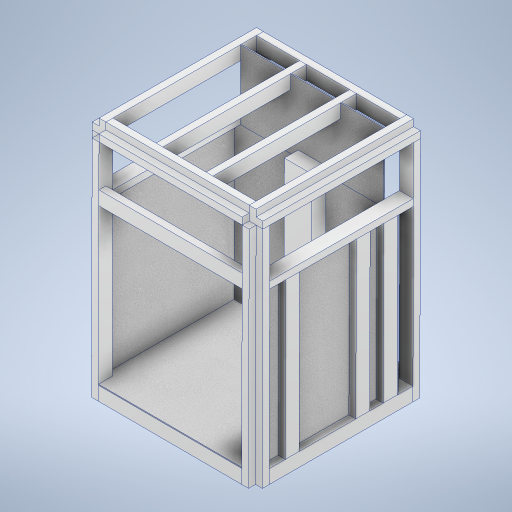
# Autodesk Inventor part: Rev IV Envelope Frame Study
Saved by Autodesk Inventor 2024 (Build 280153000, 153)
## iProperties
Created: 2024-12-08
Part Number: Rev IV Envelope Frame Study
Material: Aluminum 6061
Document SubType Name: Modeling
Designer: Ishaan
Density: 2.7 g/cm^3
Appearance: Aluminum - Flat
Author: Ishaan
Autodesk Inventor part; units mm, degrees
ref_plane "YZ Plane" through (0, 0, 0) normal (1, 0, 0) x (0, 1, 0)
ref_plane "XZ Plane" through (0, 0, 0) normal (0, 1, 0) x (-1, 0, 0)
ref_plane "XY Plane" through (0, 0, 0) normal (0, 0, 1) x (1, 0, 0)
sketch "Sketch1" plane through (0, 0, 0) normal (0, 0, 1) x (1, 0, 0)
  line L0 (247.5, -247.5) -> (-247.5, -247.5) construction
  line L1 (-247.5, -247.5) -> (-247.5, 247.5) construction
  line L2 (-247.5, 247.5) -> (247.5, 247.5) construction
  line L3 (247.5, 247.5) -> (247.5, -247.5) construction
  line L4 (247.5, -247.5) -> (-247.5, 247.5) construction
  line L5 (-247.5, -247.5) -> (247.5, 247.5) construction
  line L6 (-247.5, 247.5) -> (-207.5, 247.5)
  line L7 (-207.5, 247.5) -> (-207.5, 207.5)
  line L8 (-207.5, 207.5) -> (-247.5, 207.5)
  line L9 (-247.5, 207.5) -> (-247.5, 247.5)
  line L10 (-247.5, 247.5) -> (-227.5, 247.5)
  line L11 (-227.5, 247.5) -> (-227.5, 227.5)
  line L12 (-227.5, 227.5) -> (-247.5, 227.5)
  line L13 (-247.5, 227.5) -> (-247.5, 247.5)
  line L14 (247.5, 247.5) -> (207.5, 247.5)
  line L15 (207.5, 247.5) -> (207.5, 207.5)
  line L16 (207.5, 207.5) -> (247.5, 207.5)
  line L17 (247.5, 207.5) -> (247.5, 247.5)
  line L18 (247.5, 247.5) -> (227.5, 247.5)
  line L19 (227.5, 247.5) -> (227.5, 227.5)
  line L20 (227.5, 227.5) -> (247.5, 227.5)
  line L21 (247.5, 227.5) -> (247.5, 247.5)
  line L22 (247.5, -247.5) -> (207.5, -247.5)
  line L23 (207.5, -247.5) -> (207.5, -207.5)
  line L24 (207.5, -207.5) -> (247.5, -207.5)
  line L25 (247.5, -207.5) -> (247.5, -247.5)
  line L26 (247.5, -247.5) -> (227.5, -247.5)
  line L27 (227.5, -247.5) -> (227.5, -227.5)
  line L28 (227.5, -227.5) -> (247.5, -227.5)
  line L29 (247.5, -227.5) -> (247.5, -247.5)
  line L30 (-247.5, -247.5) -> (-207.5, -247.5)
  line L31 (-207.5, -247.5) -> (-207.5, -207.5)
  line L32 (-207.5, -207.5) -> (-247.5, -207.5)
  line L33 (-247.5, -207.5) -> (-247.5, -247.5)
  line L34 (-247.5, -247.5) -> (-227.5, -247.5)
  line L35 (-227.5, -247.5) -> (-227.5, -227.5)
  line L36 (-227.5, -227.5) -> (-247.5, -227.5)
  line L37 (-247.5, -227.5) -> (-247.5, -247.5)
  point P0 (0, 0)
  point P1 (227.5, -247.5)
  point P2 (247.5, -227.5)
  point P3 (247.5, 227.5)
  point P4 (227.5, 247.5)
  point P5 (-247.5, -227.5)
  point P6 (-227.5, -247.5)
  point P7 (-227.5, 247.5)
  point P8 (-247.5, 227.5)
  dimension "d0" = 495
  dimension "d1" = 495
  dimension "d2" = 40
  dimension "d3" = 40
  dimension "d4" = 20
  dimension "d5" = 20
  dimension "d6" = 40
  dimension "d7" = 40
  dimension "d8" = 20
  dimension "d9" = 20
  dimension "d10" = 40
  dimension "d11" = 40
  dimension "d12" = 20
  dimension "d13" = 20
  dimension "d14" = 40
  dimension "d15" = 40
  dimension "d16" = 20
  dimension "d17" = 20
  constraints: 76 end point, 18 parallel, 9 horizontal, 9 perpendicular, 2 midpoint
  measures "d0" distance of L1.end L2.end
  measures "d1" distance of L0.end L1.end
  measures "d2" distance of L7.end L8.end
  measures "d3" distance of L6.end L7.end
  measures "d4" distance of L11.end L12.end
  measures "d5" distance of L10.end L11.end
  measures "d6" distance of L16.end L15.end
  measures "d7" distance of L15.end L14.end
  measures "d8" distance of L20.end L19.end
  measures "d9" distance of L19.end L18.end
  measures "d10" distance of L23.end L24.end
  measures "d11" distance of L22.end L23.end
  measures "d12" distance of L27.end L28.end
  measures "d13" distance of L26.end L27.end
  measures "d14" distance of L32.end L31.end
  measures "d15" distance of L31.end L30.end
  measures "d16" distance of L36.end L35.end
  measures "d17" distance of L35.end L34.end
extrude "Extrusion1" add sketch "Sketch1" along normal blind 650 contours L6 L7 L8 L9 L12 L11 | L19 L20 L17 L16 L15 L14 | L22 L23 L24 L25 L28 L27 | L35 L36 L33 L32 L31 L30
sketch "Sketch2" plane through (-247.5, 227.5, 0) normal (0, 1, 0) x (1, 0, 0)
  line L0 (20, 0) -> (0, 0) projected
  line L1 (0, 0) -> (0, -650) projected
  line L2 (20, -650) -> (0, -650) projected
  line L3 (20, 0) -> (20, -650) projected
  line L4 (0, -650) -> (40, -650) projected
  line L5 (0, -650) -> (40, -650)
  line L6 (40, -650) -> (40, -690)
  line L7 (40, -690) -> (0, -690)
  line L8 (0, -690) -> (0, -650)
  line L9 (0, -690) -> (20, -690)
  line L10 (20, -690) -> (20, -670)
  line L11 (20, -670) -> (0, -670)
  line L12 (0, -670) -> (0, -690)
  line L13 (495, 0) -> (495, -650) projected
  line L14 (495, -650) -> (455, -650)
  line L15 (455, -650) -> (455, -690)
  line L16 (455, -690) -> (495, -690)
  line L17 (495, -690) -> (495, -650)
  line L18 (495, -690) -> (475, -690)
  line L19 (475, -690) -> (475, -670)
  line L20 (475, -670) -> (495, -670)
  line L21 (495, -670) -> (495, -690)
  point P0 (247.5, 0)
  point P1 (0, -670)
  dimension "d20" = 40
  dimension "d21" = 40
  dimension "d22" = 20
  dimension "d23" = 20
  dimension "d24" = 40
  dimension "d25" = 40
  dimension "d26" = 20
  dimension "d27" = 20
  constraints: 32 end point, 8 parallel, 4 horizontal, 4 perpendicular
  measures "d20" distance of L6.end L7.end
  measures "d21" distance of L5.end L6.end
  measures "d22" distance of L11.end L10.end
  measures "d23" distance of L10.end L9.end
  measures "d24" distance of L16.end L15.end
  measures "d25" distance of L15.end L14.end
  measures "d26" distance of L19.end L20.end
  measures "d27" distance of L18.end L19.end
extrude "Extrusion2" add sketch "Sketch2" against normal up to surface (455 mm away) separate body contours L4 L6 L7 L10 L11 L8 L2 | L17 L20 L19 L16 L15 L14
sketch "Sketch3" plane through (-207.5, 227.5, 690) normal (1, 0, 0) x (0, 0, -1)
  line L0 (0, -455) -> (40, -455) projected
  line L1 (40, 0) -> (40, -455) projected
  line L2 (0, 0) -> (40, 0) projected
  line L3 (0, 0) -> (0, -455) projected
  line L4 (40, -475) -> (40, -435) projected
  line L5 (40, -475) -> (0, -475)
  line L6 (0, -475) -> (0, -435)
  line L7 (0, -435) -> (40, -435)
  line L8 (40, -435) -> (40, -475)
  line L9 (0, -475) -> (20, -475)
  line L10 (20, -475) -> (20, -455)
  line L11 (20, -455) -> (0, -455)
  line L12 (0, -455) -> (0, -475)
  line L13 (40, -20) -> (40, 20) projected
  line L14 (690, 20) -> (40, 20) projected
  line L15 (40, 20) -> (0, 20)
  line L16 (0, 20) -> (0, -20)
  line L17 (0, -20) -> (40, -20)
  line L18 (40, -20) -> (40, 20)
  line L19 (0, 20) -> (20, 20)
  line L20 (20, 20) -> (20, 0)
  line L21 (20, 0) -> (0, 0)
  line L22 (0, 0) -> (0, 20)
  point P0 (690, -227.5)
  point P1 (20, -455)
  point P2 (0, -435)
  dimension "d30" = 40
  dimension "d31" = 40
  dimension "d32" = 20
  dimension "d33" = 20
  dimension "d34" = 40
  dimension "d35" = 40
  dimension "d36" = 20
  dimension "d37" = 20
  constraints: 32 end point, 8 parallel, 4 horizontal, 4 perpendicular
  measures "d30" distance of L6.end L7.end
  measures "d31" distance of L5.end L6.end
  measures "d32" distance of L11.end L10.end
  measures "d33" distance of L10.end L9.end
  measures "d34" distance of L17.end L16.end
  measures "d35" distance of L16.end L15.end
  measures "d36" distance of L20.end L21.end
  measures "d37" distance of L19.end L20.end
extrude "Extrusion3" add sketch "Sketch3" along normal up to surface (415 mm away) separate body contours L3 L7 L1 L0 | L0 L4 L5 L10 | L3 L2 L1 L17 | L20 L15 L13 L2
sketch "Sketch4" plane through (207.5, 207.5, 0) normal (0, -1, 0) x (1, 0, 0)
  line L0 (-455, 0) -> (-415, 0) projected
  line L1 (-415, 0) -> (-415, 650) projected
  line L2 (-455, 650) -> (-415, 650) projected
  line L3 (-455, 0) -> (-455, 650) projected
  line L4 (0, 0) -> (40, 0) projected
  line L5 (40, 0) -> (40, 650) projected
  line L6 (0, 650) -> (40, 650) projected
  line L7 (0, 0) -> (0, 650) projected
  line L8 (-455, 0) -> (-415, 0)
  line L9 (-415, 0) -> (-415, 40)
  line L10 (-415, 40) -> (-455, 40)
  line L11 (-455, 40) -> (-455, 0)
  line L12 (40, 0) -> (0, 0)
  line L13 (0, 0) -> (0, 40)
  line L14 (0, 40) -> (40, 40)
  line L15 (40, 40) -> (40, 0)
  point P0 (-207.5, 0)
  dimension "d40" = 40
  dimension "d41" = 40
  dimension "d42" = 40
  dimension "d43" = 40
  constraints: 16 end point, 4 parallel, 2 horizontal, 2 perpendicular
  measures "d40" distance of L10.end L9.end
  measures "d41" distance of L9.end L8.end
  measures "d42" distance of L13.end L14.end
  measures "d43" distance of L12.end L13.end
extrude "Extrusion4" add sketch "Sketch4" along normal up to surface (415 mm away) separate body contours L3 L10 L1 L0 | L7 L14 L5 L4
sketch "Sketch5" plane through (-207.5, -247.5, 0) normal (1, 0, 0) x (0, 0, -1)
  line L0 (0, 0) -> (0, 40) projected
  line L1 (-650, 0) -> (-650, 40) projected
  line L2 (0, 0) -> (-650, 0) projected
  line L3 (0, 455) -> (0, 495) projected
  line L4 (0, 495) -> (-650, 495) projected
  line L5 (-650, 455) -> (-650, 495) projected
  line L6 (0, 0) -> (-40, 0)
  line L7 (-40, 0) -> (-40, 20)
  line L8 (-40, 20) -> (0, 20)
  line L9 (0, 20) -> (0, 0)
  line L10 (0, 495) -> (-40, 495)
  line L11 (-40, 495) -> (-40, 475)
  line L12 (-40, 475) -> (0, 475)
  line L13 (0, 475) -> (0, 495)
  line L14 (-40, 455) -> (-40, 40) projected
  point P0 (0, 247.5)
  point P1 (0, 475)
  point P2 (0, 20)
  dimension "d91" = 20
  dimension "d111" = 20
  constraints: 16 end point, 4 parallel, 2 collinear, 2 horizontal, 2 perpendicular
  measures "d91" distance of L10.end L11.end
  measures "d111" distance of L6.end L7.end
extrude "Extrusion5" add sketch "Sketch5" along normal up to surface (415 mm away) separate body
sketch "Sketch6" plane through (-247.5, 207.5, 40) normal (0, 0, 1) x (1, 0, 0)
  line L0 (495, 0) -> (455, 0) projected
  line L1 (455, 0) -> (455, 40) projected
  line L2 (455, 40) -> (475, 40) projected
  line L3 (475, 40) -> (475, 20) projected
  line L4 (475, 20) -> (495, 20) projected
  line L5 (495, 20) -> (495, 0) projected
  line L6 (0, -415) -> (40, -415) projected
  line L7 (40, -435) -> (40, -455) projected
  line L8 (40, -455) -> (20, -455) projected
  line L9 (20, -455) -> (20, -435) projected
  line L10 (20, -435) -> (0, -435) projected
  line L11 (0, -435) -> (0, -415) projected
  line L12 (455, -415) -> (495, -415) projected
  line L13 (495, -415) -> (495, -435) projected
  line L14 (495, -435) -> (475, -435) projected
  line L15 (475, -435) -> (475, -455) projected
  line L16 (475, -455) -> (455, -455) projected
  line L17 (455, -455) -> (455, -415) projected
  line L18 (40, 0) -> (0, 0) projected
  line L19 (0, 0) -> (0, 20) projected
  line L20 (0, 20) -> (20, 20) projected
  line L21 (20, 20) -> (20, 40) projected
  line L22 (20, 40) -> (40, 40) projected
  line L23 (40, 40) -> (40, 20) projected
  line L24 (455, -415) -> (455, 0) projected
  line L25 (455, 0) -> (495, 0) projected
  line L26 (495, 0) -> (495, -415) projected
  line L27 (495, -415) -> (455, -415) projected
  line L28 (0, 0) -> (40, 0) projected
  line L29 (40, 20) -> (40, -435) projected
  line L30 (40, -415) -> (0, -415) projected
  line L31 (0, -415) -> (0, 0) projected
  line L32 (455, 20) -> (40, 20) projected
  line L33 (40, 20) -> (40, 40) projected
  line L34 (40, 40) -> (455, 40) projected
  line L35 (455, 40) -> (455, 20) projected
  line L36 (40, -455) -> (40, -435) projected
  line L37 (40, -435) -> (455, -435) projected
  line L38 (455, -435) -> (455, -455) projected
  line L39 (455, -455) -> (40, -455) projected
  line L40 (0, -369) -> (20, -369)
  line L41 (20, -369) -> (20, -329)
  line L42 (20, -329) -> (0, -329)
  line L43 (0, -329) -> (0, -369)
  line L44 (20, -165) -> (0, -165)
  line L45 (0, -165) -> (0, -125)
  line L46 (0, -125) -> (20, -125)
  line L47 (20, -125) -> (20, -165)
  line L48 (0, -46) -> (20, -46)
  line L49 (20, -46) -> (20, -86)
  line L50 (20, -86) -> (0, -86)
  line L51 (0, -86) -> (0, -46)
  line L52 (10, -165) -> (10, -329) construction
  point P0 (247.5, -207.5)
  point P1 (0, -369)
  point P2 (0, -46)
  point P3 (10, -247)
  dimension "d48" = 20
  dimension "d49" = 40
  dimension "d50" = 20
  dimension "d51" = 40
  dimension "d52" = 20
  dimension "d53" = 40
  dimension "d54" = 86
  dimension "d57" = 86
  dimension "d128" = 208
  dimension "d129" = 164
  constraints: 26 end point, 6 parallel, 3 horizontal, 3 midpoint, 3 perpendicular, 2 point on line, 1 collinear
  measures "d48" distance of L42.end L41.end
  measures "d49" distance of L41.end L40.end
  measures "d50" distance of L45.end L46.end
  measures "d51" distance of L44.end L45.end
  measures "d52" distance of L49.end L50.end
  measures "d53" distance of L48.end L49.end
  measures "d54" distance between parallel lines of L42 L6
  measures "d57" distance between parallel lines of L28 L50
  measures "d128" distance from line of L39 point (10, -247)
  measures "d129" distance of L52.start L52.end
extrude "Extrusion6" add sketch "Sketch6" along normal blind 450 separate body contours L48 L49 L50 L31 | L31 L42 L41 L40 | L46 L47 L44 L31
mirror "Mirror1" about plane through (0, 0, 0) normal (1, 0, 0) of "Extrusion6" bodies 6
sketch "Sketch7" plane through (-247.5, 207.5, 0) normal (0, -1, 0) x (1, 0, 0)
  line L0 (0, 0) -> (40, 0) projected
  line L1 (40, 0) -> (40, 650) projected
  line L2 (0, 650) -> (40, 650) projected
  line L3 (0, 0) -> (0, 650) projected
  line L4 (455, 0) -> (495, 0) projected
  line L5 (495, 0) -> (495, 650) projected
  line L6 (455, 650) -> (495, 650) projected
  line L7 (455, 0) -> (455, 650) projected
  line L8 (0, 490) -> (40, 490)
  line L9 (40, 490) -> (40, 510)
  line L10 (40, 510) -> (0, 510)
  line L11 (0, 510) -> (0, 490)
  line L12 (495, 490) -> (455, 490)
  line L13 (455, 490) -> (455, 510)
  line L14 (455, 510) -> (495, 510)
  line L15 (495, 510) -> (495, 490)
  line L16 (40, 0) -> (40, 650) projected
  point P0 (247.5, 0)
  point P1 (0, 510)
  dimension "d60" = 20
  constraints: 16 end point, 4 parallel, 2 collinear, 2 horizontal, 2 perpendicular, 1 point on line
  measures "d60" distance of L9.end L8.end
extrude "Extrusion7" add sketch "Sketch7" along normal up to surface (415 mm away) separate body contours L3 L10 L1 L8 | L7 L14 L5 L12
sketch "Sketch8" plane through (-207.5, -247.5, 0) normal (1, 0, 0) x (0, 0, -1)
  line L0 (0, 0) -> (0, 40) projected
  line L1 (0, 40) -> (-650, 40) projected
  line L2 (-650, 0) -> (-650, 40) projected
  line L3 (0, 0) -> (-650, 0) projected
  line L4 (0, 0) -> (-650, 0) projected
  line L5 (-490, 0) -> (-530, 0)
  line L6 (-530, 0) -> (-530, 20)
  line L7 (-530, 20) -> (-490, 20)
  line L8 (-490, 20) -> (-490, 0)
  line L9 (-490, 455) -> (-490, 40) projected
  point P0 (0, 247.5)
  dimension "d64" = 40
  dimension "d65" = 20
  constraints: 8 end point, 2 parallel, 1 collinear, 1 horizontal, 1 perpendicular, 1 point on line
  measures "d64" distance of L6.end L7.end
  measures "d65" distance of L5.end L6.end
extrude "Extrusion8" add sketch "Sketch8" along normal up to surface (415 mm away) separate body contours L3 L6 L7 L8
sketch "Sketch12" plane through (-227.5, -161.5, 40) normal (1, 0, 0) x (0, 0, -1)
  line L0 (-450, 369) -> (-450, -46) projected
  line L1 (0, 323) -> (-450, 323) projected
  line L2 (0, 283) -> (0, 323) projected
  line L3 (0, 323) -> (-450, 323)
  line L4 (-450, 323) -> (-450, -46)
  line L5 (-450, -46) -> (0, -46)
  line L6 (0, -46) -> (0, 323)
  point P0 (40, 161.5)
  constraints: 8 end point, 2 parallel, 1 horizontal, 1 perpendicular
extrude "Extrusion12" add sketch "Sketch12" along normal blind 3 separate body
mirror "Mirror2" about plane through (0, 0, 0) normal (1, 0, 0) of "Extrusion12" bodies 9
sketch "Sketch16" plane through (-207.5, 227.5, 40) normal (0, 0, 1) x (1, 0, 0)
  line L0 (415, 20) -> (415, 0) projected
  line L1 (0, 20) -> (415, 20) projected
  line L2 (0, 20) -> (0, 0) projected
  line L3 (0, 0) -> (415, 0) projected
  line L4 (290, -23) -> (270, -23)
  line L5 (270, -23) -> (270, -63)
  line L6 (270, -63) -> (290, -63)
  line L7 (290, -63) -> (290, -23)
  line L8 (145, -23) -> (125, -23)
  line L9 (125, -23) -> (125, -63)
  line L10 (125, -63) -> (145, -63)
  line L11 (145, -63) -> (145, -23)
  line L12 (270, -43) -> (145, -43) construction
  point P0 (207.5, -227.5)
  point P1 (207.5, -43)
  point P2 (125, 20)
  point P3 (270, 20)
  point P4 (125, 0)
  point P5 (145, 0)
  point P6 (270, 0)
  point P7 (290, 0)
  dimension "d99" = 20
  dimension "d100" = 40
  dimension "d101" = 20
  dimension "d102" = 40
  dimension "d103" = 125
  dimension "d104" = 125
  dimension "d127" = 83
  constraints: 18 end point, 4 parallel, 3 midpoint, 2 horizontal, 2 perpendicular, 1 collinear, 1 vertical alignment
  measures "d99" distance of L6.end L5.end
  measures "d100" distance of L5.end L4.end
  measures "d101" distance of L10.end L9.end
  measures "d102" distance of L9.end L8.end
  measures "d103" distance of L12.start L12.end
  measures "d104" distance between parallel lines of L0 L7
  measures "d127" distance between parallel lines of L6 L1
extrude "Extrusion16" add sketch "Sketch16" along normal up to surface (610 mm away) separate body contours L7 L6 L5 L4 | L11 L10 L9 L8
sketch "Sketch17" plane through (-207.5, 207.5, 650) normal (0, -1, 0) x (1, 0, 0)
  line L0 (125, 0) -> (145, 0) projected
  line L1 (270, 0) -> (290, 0) projected
  line L2 (415, 40) -> (415, 0) projected
  line L3 (0, 40) -> (415, 40) projected
  line L4 (0, 40) -> (0, 0) projected
  line L5 (0, 0) -> (415, 0) projected
  line L6 (125, 0) -> (145, 0)
  line L7 (145, 0) -> (145, 40)
  line L8 (145, 40) -> (125, 40)
  line L9 (125, 40) -> (125, 0)
  line L10 (290, 0) -> (270, 0)
  line L11 (270, 0) -> (270, 40)
  line L12 (270, 40) -> (290, 40)
  line L13 (290, 40) -> (290, 0)
  point P0 (207.5, -650)
  point P1 (290, 40)
  point P2 (125, 40)
  constraints: 16 end point, 4 parallel, 4 point on line, 2 horizontal, 2 perpendicular
extrude "Extrusion17" add sketch "Sketch17" along normal up to surface (415 mm away) separate body contours L9 L3 L7 L0 | L11 L3 L13 L1
sketch "Sketch18" plane through (-207.5, 227.5, 0) normal (0, -1, 0) x (1, 0, 0)
  line L0 (125, 40) -> (145, 40) projected
  line L1 (145, 40) -> (125, 40) projected
  line L2 (290, 40) -> (270, 40) projected
  line L3 (270, 40) -> (290, 40) projected
  line L4 (0, 0) -> (415, 0) projected
  line L5 (125, 40) -> (145, 40)
  line L6 (145, 40) -> (145, 0)
  line L7 (145, 0) -> (125, 0)
  line L8 (125, 0) -> (125, 40)
  line L9 (290, 40) -> (270, 40)
  line L10 (270, 40) -> (270, 0)
  line L11 (270, 0) -> (290, 0)
  line L12 (290, 0) -> (290, 40)
  point P0 (207.5, 0)
  point P1 (270, 0)
  point P2 (125, 40)
  point P3 (125, 0)
  point P4 (145, 40)
  constraints: 16 end point, 4 parallel, 4 point on line, 2 horizontal, 2 perpendicular
extrude "Extrusion18" add sketch "Sketch18" along normal up to surface (455 mm away) separate body
sketch "Sketch19" plane through (-247.5, 161.5, 40) normal (0, 1, 0) x (1, 0, 0)
  line L0 (455, -610) -> (495, -610) projected
  line L1 (495, -610) -> (495, -630) projected
  line L2 (495, -630) -> (475, -630) projected
  line L3 (475, -630) -> (475, -650) projected
  line L4 (475, -650) -> (455, -650) projected
  line L5 (455, -650) -> (455, -610) projected
  line L6 (20, -650) -> (20, -630) projected
  line L7 (20, -630) -> (0, -630) projected
  line L8 (0, -630) -> (0, -610) projected
  line L9 (0, -610) -> (40, -610) projected
  line L10 (40, -610) -> (40, -650) projected
  line L11 (40, -650) -> (20, -650) projected
  line L12 (455, 0) -> (455, 40) projected
  line L13 (455, 40) -> (495, 40) projected
  line L14 (495, 40) -> (495, 0) projected
  line L15 (495, 0) -> (455, 0) projected
  line L16 (0, 40) -> (40, 40) projected
  line L17 (40, 40) -> (40, 0) projected
  line L18 (40, 0) -> (0, 0) projected
  line L19 (0, 0) -> (0, 40) projected
  line L20 (0, -450) -> (0, 0) projected
  line L21 (0, 0) -> (20, 0) projected
  line L22 (20, 0) -> (20, -450) projected
  line L23 (20, -450) -> (0, -450) projected
  line L24 (495, 0) -> (495, -450) projected
  line L25 (495, -450) -> (475, -450) projected
  line L26 (475, -450) -> (475, 0) projected
  line L27 (475, 0) -> (495, 0) projected
  line L28 (455, -470) -> (455, -450) projected
  line L29 (455, -450) -> (495, -450) projected
  line L30 (495, -450) -> (495, -470) projected
  line L31 (495, -470) -> (455, -470) projected
  line L32 (0, -450) -> (40, -450) projected
  line L33 (40, -450) -> (40, -470) projected
  line L34 (40, -470) -> (0, -470) projected
  line L35 (0, -470) -> (0, -450) projected
  line L36 (23, -450) -> (20, -450) projected
  line L37 (20, -450) -> (20, 0) projected
  line L38 (20, 0) -> (23, 0) projected
  line L39 (23, 0) -> (23, -450) projected
  line L40 (475, -450) -> (472, -450) projected
  line L41 (472, -450) -> (472, 0) projected
  line L42 (472, 0) -> (475, 0) projected
  line L43 (475, 0) -> (475, -450) projected
  line L44 (330, -650) -> (310, -650) projected
  line L45 (310, -650) -> (310, -610) projected
  line L46 (310, -610) -> (330, -610) projected
  line L47 (330, -610) -> (330, -650) projected
  line L48 (185, -610) -> (185, -650) projected
  line L49 (185, -650) -> (165, -650) projected
  line L50 (165, -650) -> (165, -610) projected
  line L51 (165, -610) -> (185, -610) projected
  line L52 (330, 0) -> (310, 0) projected
  line L53 (310, 0) -> (310, 40) projected
  line L54 (310, 40) -> (330, 40) projected
  line L55 (330, 40) -> (330, 0) projected
  line L56 (185, 40) -> (185, 0) projected
  line L57 (185, 0) -> (165, 0) projected
  line L58 (165, 0) -> (165, 40) projected
  line L59 (165, 40) -> (185, 40) projected
  line L60 (495, 0) -> (0, 0)
  line L61 (0, 0) -> (0, -450)
  line L62 (0, -450) -> (495, -450)
  line L63 (495, -450) -> (495, 0)
  point P0 (247.5, 40)
  point P1 (330, 0)
  point P2 (310, 0)
  point P3 (185, 0)
  point P4 (165, 0)
  constraints: 8 end point, 2 parallel, 1 horizontal, 1 perpendicular
extrude "Extrusion19" add sketch "Sketch19" along normal blind 3 separate body contours L15 L41 L29 L62 L32 L39 L18 L60 L57 L52 | L15 L26 L29 L41 | L15 L24 L25 L26 | L32 L22 L18 L39 | L23 L20 L18 L22
sketch "Sketch23" plane through (-82.5, 227.5, 40) normal (0, 0, 1) x (1, 0, 0)
  line L0 (330, -66) -> (-165, -66) projected
  line L1 (20, -455) -> (0, -455) projected
  line L2 (20, 0) -> (20, -455) projected
  line L3 (20, 0) -> (0, 0) projected
  line L4 (0, 0) -> (0, -455) projected
  line L5 (165, -455) -> (145, -455) projected
  line L6 (165, 0) -> (165, -455) projected
  line L7 (165, 0) -> (145, 0) projected
  line L8 (145, 0) -> (145, -455) projected
  line L9 (145, 0) -> (145, -455) projected
  line L10 (20, -66) -> (145, -66)
  line L11 (145, -66) -> (145, -106)
  line L12 (145, -106) -> (20, -106)
  line L13 (20, -106) -> (20, -66)
  line L14 (42.5, -106) -> (122.5, -106)
  line L15 (122.5, -106) -> (122.5, -66)
  line L16 (122.5, -66) -> (42.5, -66)
  line L17 (42.5, -66) -> (42.5, -106)
  point P0 (82.5, -227.5)
  point P1 (82.5, -106)
  point P2 (145, -66)
  point P3 (42.5, -66)
  point P4 (42.5, -106)
  dimension "d130" = 40
  dimension "d131" = 80
  constraints: 16 end point, 4 parallel, 3 point on line, 2 horizontal, 2 midpoint, 2 perpendicular, 1 collinear
  measures "d130" distance of L10.end L11.end
  measures "d131" distance of L16.end L15.end
extrude "Extrusion23" add sketch "Sketch23" against normal blind 20 separate body contours L8 L12 L15 L0 | L15 L12 L17 L0 | L17 L12 L2 L0
extrude "Extrusion24" add sketch "Sketch23" along normal blind 470 separate body contours L15 L12 L17 L0
sketch "Sketch24" plane through (62.5, 164.5, 40) normal (-1, 0, 0) x (0, 0, 1)
  line L0 (470, -43) -> (470, -3) projected
  line L1 (470, -3) -> (470, -43) projected
  line L2 (610, 40) -> (610, 0) projected
  line L3 (0, 40) -> (610, 40) projected
  line L4 (0, 40) -> (0, 0) projected
  line L5 (0, 0) -> (610, 0) projected
  line L6 (0, 0) -> (610, 0) projected
  line L7 (470, 0) -> (450, 0)
  line L8 (450, 0) -> (450, 40)
  line L9 (450, 40) -> (470, 40)
  line L10 (470, 40) -> (470, 0)
  point P0 (-40, -164.5)
  point P1 (470, 0)
  point P2 (470, 40)
  point P3 (450, 0)
  dimension "d136" = 20
  constraints: 8 end point, 2 parallel, 2 point on line, 1 collinear, 1 horizontal, 1 perpendicular
  measures "d136" distance of L8.end L9.end
extrude "Extrusion25" add sketch "Sketch24" along normal up to surface (125 mm away) separate body contours L10 L5 L8 L3
sketch "Sketch20" plane through (-247.5, 161.5, 40) normal (0, -1, 0) x (1, 0, 0)
  line L0 (495, 610) -> (455, 610) projected
  line L1 (455, 610) -> (455, 650) projected
  line L2 (455, 650) -> (475, 650) projected
  line L3 (475, 650) -> (475, 630) projected
  line L4 (475, 630) -> (495, 630) projected
  line L5 (495, 630) -> (495, 610) projected
  line L6 (20, 630) -> (20, 650) projected
  line L7 (20, 650) -> (40, 650) projected
  line L8 (40, 650) -> (40, 610) projected
  line L9 (40, 610) -> (0, 610) projected
  line L10 (0, 610) -> (0, 630) projected
  line L11 (0, 630) -> (20, 630) projected
  line L12 (455, -40) -> (455, 0) projected
  line L13 (455, 0) -> (495, 0) projected
  line L14 (495, 0) -> (495, -40) projected
  line L15 (495, -40) -> (455, -40) projected
  line L16 (40, -40) -> (0, -40) projected
  line L17 (0, -40) -> (0, 0) projected
  line L18 (0, 0) -> (40, 0) projected
  line L19 (40, 0) -> (40, -40) projected
  line L20 (0, 0) -> (0, 450) projected
  line L21 (0, 450) -> (20, 450) projected
  line L22 (20, 450) -> (20, 0) projected
  line L23 (20, 0) -> (0, 0) projected
  line L24 (495, 450) -> (495, 0) projected
  line L25 (495, 0) -> (475, 0) projected
  line L26 (475, 0) -> (475, 450) projected
  line L27 (475, 450) -> (495, 450) projected
  line L28 (455, 450) -> (455, 470) projected
  line L29 (455, 470) -> (495, 470) projected
  line L30 (495, 470) -> (495, 450) projected
  line L31 (495, 450) -> (455, 450) projected
  line L32 (40, 450) -> (0, 450) projected
  line L33 (0, 450) -> (0, 470) projected
  line L34 (0, 470) -> (40, 470) projected
  line L35 (40, 470) -> (40, 450) projected
  line L36 (20, 450) -> (23, 450) projected
  line L37 (23, 450) -> (23, 0) projected
  line L38 (23, 0) -> (20, 0) projected
  line L39 (20, 0) -> (20, 450) projected
  line L40 (472, 450) -> (475, 450) projected
  line L41 (475, 450) -> (475, 0) projected
  line L42 (475, 0) -> (472, 0) projected
  line L43 (472, 0) -> (472, 450) projected
  line L44 (310, 650) -> (330, 650) projected
  line L45 (330, 650) -> (330, 610) projected
  line L46 (330, 610) -> (310, 610) projected
  line L47 (310, 610) -> (310, 650) projected
  line L48 (185, 650) -> (185, 610) projected
  line L49 (185, 610) -> (165, 610) projected
  line L50 (165, 610) -> (165, 650) projected
  line L51 (165, 650) -> (185, 650) projected
  line L52 (310, 0) -> (330, 0) projected
  line L53 (330, 0) -> (330, -40) projected
  line L54 (330, -40) -> (310, -40) projected
  line L55 (310, -40) -> (310, 0) projected
  line L56 (185, 0) -> (185, -40) projected
  line L57 (185, -40) -> (165, -40) projected
  line L58 (165, -40) -> (165, 0) projected
  line L59 (165, 0) -> (185, 0) projected
  line L60 (40, 650) -> (165, 650)
  line L61 (165, 650) -> (165, 610)
  line L62 (165, 610) -> (40, 610)
  line L63 (40, 610) -> (40, 650)
  line L64 (185, 650) -> (310, 650)
  line L65 (310, 650) -> (310, 610)
  line L66 (310, 610) -> (185, 610)
  line L67 (185, 610) -> (185, 650)
  line L68 (330, 650) -> (455, 650)
  line L69 (455, 650) -> (455, 610)
  line L70 (455, 610) -> (330, 610)
  line L71 (330, 610) -> (330, 650)
  line L72 (0, -40) -> (0, 610) projected
  line L73 (40, 450) -> (455, 450)
  line L74 (455, 450) -> (455, 610)
  line L75 (455, 610) -> (40, 610)
  line L76 (40, 610) -> (40, 450)
  line L77 (495, 450) -> (495, 0) projected
  line L78 (0, 0) -> (0, 450) projected
  line L79 (0, 450) -> (495, 450) projected
  line L80 (495, 0) -> (0, 0) projected
  line L81 (310, 0) -> (310, -20) projected
  line L82 (310, -20) -> (185, -20) projected
  line L83 (185, -20) -> (185, 0) projected
  line L84 (185, 0) -> (310, 0) projected
  line L85 (207.5, 0) -> (207.5, 470) projected
  line L86 (207.5, 470) -> (287.5, 470) projected
  line L87 (287.5, 470) -> (287.5, 0) projected
  line L88 (287.5, 0) -> (207.5, 0) projected
  point P0 (247.5, -40)
  point P1 (0, 510)
  constraints: 32 end point, 8 parallel, 4 horizontal, 4 perpendicular, 2 collinear, 1 point on line, 2 other
extrude "Extrusion20" add sketch "Sketch20" against normal blind 3 separate body contours L70 L45 L68 L1 | L74 L28 L73 L87 L86 L85 L35 L76 L62 L49 L66 L46 L70 | L66 L48 L64 L47 | L73 L85 L86 L87 | L62 L8 L60 L50
sketch "Sketch22" plane through (-247.5, 207.5, 40) normal (0, 0, 1) x (1, 0, 0)
  line L0 (495, 0) -> (455, 0) projected
  line L1 (455, 20) -> (455, 40) projected
  line L2 (455, 40) -> (475, 40) projected
  line L3 (475, 40) -> (475, 20) projected
  line L4 (475, 20) -> (495, 20) projected
  line L5 (495, 20) -> (495, 0) projected
  line L6 (0, -415) -> (40, -415) projected
  line L7 (40, -435) -> (40, -455) projected
  line L8 (40, -455) -> (20, -455) projected
  line L9 (20, -455) -> (20, -435) projected
  line L10 (20, -435) -> (0, -435) projected
  line L11 (0, -435) -> (0, -415) projected
  line L12 (455, -415) -> (495, -415) projected
  line L13 (495, -415) -> (495, -435) projected
  line L14 (495, -435) -> (475, -435) projected
  line L15 (475, -435) -> (475, -455) projected
  line L16 (475, -455) -> (455, -455) projected
  line L17 (455, -455) -> (455, -435) projected
  line L18 (40, 0) -> (0, 0) projected
  line L19 (0, 0) -> (0, 20) projected
  line L20 (0, 20) -> (20, 20) projected
  line L21 (20, 20) -> (20, 40) projected
  line L22 (20, 40) -> (40, 40) projected
  line L23 (40, 40) -> (40, 20) projected
  line L24 (455, -435) -> (455, 20) projected
  line L25 (455, 0) -> (495, 0) projected
  line L26 (495, 0) -> (495, -415) projected
  line L27 (495, -415) -> (455, -415) projected
  line L28 (0, 0) -> (40, 0) projected
  line L29 (40, 20) -> (40, -435) projected
  line L30 (40, -415) -> (0, -415) projected
  line L31 (0, -415) -> (0, 0) projected
  line L32 (455, 20) -> (40, 20) projected
  line L33 (40, 20) -> (40, 40) projected
  line L34 (40, 40) -> (455, 40) projected
  line L35 (455, 40) -> (455, 20) projected
  line L36 (40, -455) -> (40, -435) projected
  line L37 (40, -435) -> (455, -435) projected
  line L38 (455, -435) -> (455, -455) projected
  line L39 (455, -455) -> (40, -455) projected
  line L40 (20, -46) -> (20, -86) projected
  line L41 (20, -86) -> (0, -86) projected
  line L42 (0, -86) -> (0, -46) projected
  line L43 (0, -46) -> (20, -46) projected
  line L44 (20, -125) -> (20, -165) projected
  line L45 (20, -165) -> (0, -165) projected
  line L46 (0, -165) -> (0, -125) projected
  line L47 (0, -125) -> (20, -125) projected
  line L48 (20, -329) -> (20, -369) projected
  line L49 (20, -369) -> (0, -369) projected
  line L50 (0, -369) -> (0, -329) projected
  line L51 (0, -329) -> (20, -329) projected
  line L52 (475, -86) -> (475, -46) projected
  line L53 (475, -46) -> (495, -46) projected
  line L54 (495, -46) -> (495, -86) projected
  line L55 (495, -86) -> (475, -86) projected
  line L56 (475, -165) -> (475, -125) projected
  line L57 (475, -125) -> (495, -125) projected
  line L58 (495, -125) -> (495, -165) projected
  line L59 (495, -165) -> (475, -165) projected
  line L60 (475, -369) -> (475, -329) projected
  line L61 (475, -329) -> (495, -329) projected
  line L62 (495, -329) -> (495, -369) projected
  line L63 (495, -369) -> (475, -369) projected
  line L64 (20, -46) -> (23, -46) projected
  line L65 (23, -46) -> (23, -415) projected
  line L66 (23, -415) -> (20, -415) projected
  line L67 (20, -415) -> (20, -46) projected
  line L68 (472, -46) -> (475, -46) projected
  line L69 (475, -46) -> (475, -415) projected
  line L70 (475, -415) -> (472, -415) projected
  line L71 (472, -415) -> (472, -46) projected
  line L72 (165, -43) -> (165, -3) projected
  line L73 (165, -3) -> (185, -3) projected
  line L74 (185, -3) -> (185, -43) projected
  line L75 (185, -43) -> (165, -43) projected
  line L76 (310, -43) -> (310, -3) projected
  line L77 (310, -3) -> (330, -3) projected
  line L78 (330, -3) -> (330, -43) projected
  line L79 (330, -43) -> (310, -43) projected
  line L80 (330, -435) -> (310, -435) projected
  line L81 (310, -435) -> (310, 20) projected
  line L82 (310, 20) -> (330, 20) projected
  line L83 (330, 20) -> (330, -435) projected
  line L84 (165, 20) -> (185, 20) projected
  line L85 (185, 20) -> (185, -435) projected
  line L86 (185, -435) -> (165, -435) projected
  line L87 (165, -435) -> (165, 20) projected
  line L88 (0, -46) -> (0, -43) projected
  line L89 (0, -43) -> (495, -43) projected
  line L90 (495, -43) -> (495, -46) projected
  line L91 (495, -46) -> (0, -46) projected
  line L92 (23, -46) -> (472, -46)
  line L93 (472, -46) -> (472, -415)
  line L94 (472, -415) -> (23, -415)
  line L95 (23, -415) -> (23, -46)
  line L96 (455, -435) -> (40, -435)
  line L97 (40, -435) -> (40, -455)
  line L98 (40, -455) -> (455, -455)
  line L99 (455, -455) -> (455, -435)
  line L100 (310, -86) -> (185, -86) projected
  line L101 (185, -86) -> (185, -46) projected
  line L102 (185, -46) -> (310, -46) projected
  line L103 (310, -46) -> (310, -86) projected
  line L104 (207.5, -86) -> (207.5, -46) projected
  line L105 (207.5, -46) -> (287.5, -46) projected
  line L106 (287.5, -46) -> (287.5, -86) projected
  line L107 (287.5, -86) -> (207.5, -86) projected
  point P0 (247.5, -207.5)
  point P1 (40, -415)
  point P2 (455, -415)
  constraints: 16 end point, 4 parallel, 2 horizontal, 2 perpendicular, 4 other
extrude "Extrusion22" add sketch "Sketch22" along normal blind 3 separate body contours L91 L71 L12 L24 | L24 L94 L83 L91 | L24 L37 L83 L94 | L83 L94 L81 L91 | L17 L39 L7 L37 | L83 L37 L81 L94 | L81 L100 L106 L91 | L94 L85 L100 L81 | L81 L37 L85 L94 | L91 L104 L100 L85 | L85 L94 L87 L91 | L85 L37 L87 L94 | L87 L94 L29 L91 | L29 L6 L65 L91 | L29 L94 L87 L37
equation "\"d43\" = d41"
equation "\"d54\" = d57"
equation "\"d102\" = d100"
body "Solid1"
body "Solid2"
body "Solid3"
body "Solid4"
body "Solid5"
body "Solid6"
body "Solid7"
body "Solid8"
body "Solid12"
body "Solid16"
body "Solid17"
body "Solid18"
body "Solid19"
body "Solid20"
body "Solid22"
body "Solid23"
body "Solid24"
body "Solid25"
